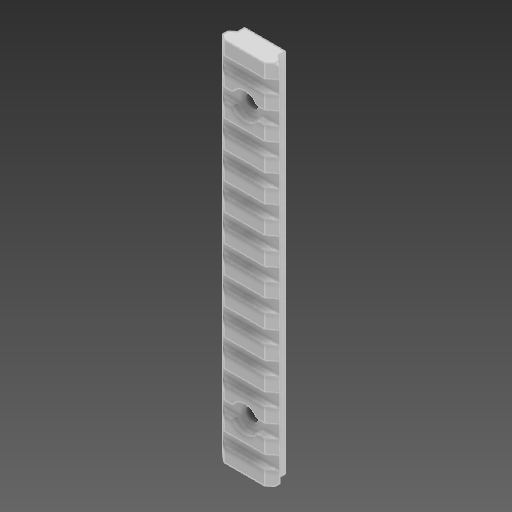
# Autodesk Inventor part: Picatinny14
Saved by Autodesk Inventor 2020.4 (Build 244396010, 396A)
## iProperties
Created: 2022-09-17
Part Number: Picatinny14
Material: Generic
Document SubType Name: Modeling
Designer: Val
Density: 1 g/cm^3
Appearance: Default
Author: Val
Autodesk Inventor part; units mm, degrees
ref_plane "YZ Plane" through (0, 0, 0) normal (1, 0, 0) x (0, 1, 0)
ref_plane "XZ Plane" through (0, 0, 0) normal (0, 1, 0) x (-1, 0, 0)
ref_plane "XY Plane" through (0, 0, 0) normal (0, 0, 1) x (1, 0, 0)
sketch "Base" plane through (0, 0, 0) normal (0, 0, 1) x (1, 0, 0)
  line L0 (-7.5, 135) -> (7.5, 135)
  line L1 (7.5, 135) -> (7.5, 0)
  line L2 (7.5, 0) -> (-7.5, 0)
  line L3 (-7.5, 0) -> (-7.5, 135)
  point P0 (0, 0)
  point P1 (0, 0)
  dimension "d0" = 135
  dimension "d1" = 15
  constraints: 8 end point, 2 parallel, 1 coincident, 1 horizontal, 1 midpoint, 1 perpendicular
  measures "d0" distance of L2.end L0.start
  measures "d1" distance of L0.start L0.end
extrude "BaseFeature" add sketch "Base" along normal blind 2.54
sketch "Profile" plane through (-7.5, 0, 0) normal (0, -1, 0) x (1, 0, 0)
  line L0 (0, 2.54) -> (15, 2.54) projected
  line L1 (0, 2.54) -> (15, 2.54)
  line L2 (15, 2.54) -> (15, 7.5692) construction
  line L3 (15, 7.5692) -> (0, 7.5692)
  line L4 (0, 7.5692) -> (0, 2.54) construction
  line L5 (-3.041, 5.0546) -> (18.041, 5.0546) construction
  line L6 (15, 7.5692) -> (18.041, 5.0546)
  line L7 (15, 2.54) -> (18.041, 5.0546)
  line L8 (0, 7.5692) -> (-3.041, 5.0546)
  line L9 (-3.041, 5.0546) -> (0, 2.54)
  point P0 (7.5, 0)
  point P1 (15, 5.0546)
  dimension "d4" = 5.0292
  dimension "d5" = 21.082
  constraints: 18 end point, 4 parallel, 2 horizontal, 1 midpoint, 1 perpendicular, 1 point on line
  measures "d4" distance of L0.end L2.end
  measures "d5" distance of L5.start L5.end
extrude "ProfileFeature" add sketch "Profile" against normal up to surface (135 mm away)
sketch "Rails" plane through (-7.5, 0, 7.5692) normal (0, 0, 1) x (1, 0, 0)
  line L0 (-3.041, 0) -> (-3.041, 135) projected
  line L1 (-3.041, 135) -> (18.041, 135)
  line L2 (18.041, 135) -> (18.041, 130)
  line L3 (18.041, 130) -> (-3.041, 130)
  line L4 (-3.041, 130) -> (-3.041, 135)
  line L5 (18.041, 0) -> (18.041, 135) projected
  line L6 (18.041, 120) -> (-3.041, 120)
  line L7 (-3.041, 125) -> (18.041, 125)
  line L8 (-3.041, 120) -> (-3.041, 125)
  line L9 (18.041, 125) -> (18.041, 120)
  line L10 (18.041, 110) -> (-3.041, 110)
  line L11 (-3.041, 115) -> (18.041, 115)
  line L12 (-3.041, 110) -> (-3.041, 115)
  line L13 (18.041, 115) -> (18.041, 110)
  line L14 (18.041, 100) -> (-3.041, 100)
  line L15 (-3.041, 105) -> (18.041, 105)
  line L16 (-3.041, 100) -> (-3.041, 105)
  line L17 (18.041, 105) -> (18.041, 100)
  line L18 (18.041, 90) -> (-3.041, 90)
  line L19 (-3.041, 95) -> (18.041, 95)
  line L20 (-3.041, 90) -> (-3.041, 95)
  line L21 (18.041, 95) -> (18.041, 90)
  line L22 (18.041, 80) -> (-3.041, 80)
  line L23 (-3.041, 85) -> (18.041, 85)
  line L24 (-3.041, 80) -> (-3.041, 85)
  line L25 (18.041, 85) -> (18.041, 80)
  line L26 (18.041, 70) -> (-3.041, 70)
  line L27 (-3.041, 75) -> (18.041, 75)
  line L28 (-3.041, 70) -> (-3.041, 75)
  line L29 (18.041, 75) -> (18.041, 70)
  line L30 (18.041, 60) -> (-3.041, 60)
  line L31 (-3.041, 65) -> (18.041, 65)
  line L32 (-3.041, 60) -> (-3.041, 65)
  line L33 (18.041, 65) -> (18.041, 60)
  line L34 (18.041, 50) -> (-3.041, 50)
  line L35 (-3.041, 55) -> (18.041, 55)
  line L36 (-3.041, 50) -> (-3.041, 55)
  line L37 (18.041, 55) -> (18.041, 50)
  line L38 (18.041, 40) -> (-3.041, 40)
  line L39 (-3.041, 45) -> (18.041, 45)
  line L40 (-3.041, 40) -> (-3.041, 45)
  line L41 (18.041, 45) -> (18.041, 40)
  line L42 (18.041, 30) -> (-3.041, 30)
  line L43 (-3.041, 35) -> (18.041, 35)
  line L44 (-3.041, 30) -> (-3.041, 35)
  line L45 (18.041, 35) -> (18.041, 30)
  line L46 (18.041, 20) -> (-3.041, 20)
  line L47 (-3.041, 25) -> (18.041, 25)
  line L48 (-3.041, 20) -> (-3.041, 25)
  line L49 (18.041, 25) -> (18.041, 20)
  line L50 (18.041, 10) -> (-3.041, 10)
  line L51 (-3.041, 15) -> (18.041, 15)
  line L52 (-3.041, 10) -> (-3.041, 15)
  line L53 (18.041, 15) -> (18.041, 10)
  line L54 (18.041, 0) -> (-3.041, 0)
  line L55 (-3.041, 5) -> (18.041, 5)
  line L56 (-3.041, 0) -> (-3.041, 5)
  line L57 (18.041, 5) -> (18.041, 0)
  point P0 (7.5, 0)
  point P1 (-3.041, 10)
  point P2 (-3.041, 20)
  point P3 (18.041, 25)
  point P4 (-3.041, 30)
  point P5 (18.041, 35)
  point P6 (18.041, 40)
  point P7 (-3.041, 40)
  point P8 (-3.041, 50)
  point P9 (-3.041, 60)
  point P10 (-3.041, 70)
  point P11 (18.041, 80)
  point P12 (-3.041, 80)
  point P13 (18.041, 85)
  point P14 (18.041, 90)
  point P15 (-3.041, 90)
  point P16 (18.041, 95)
  point P17 (18.041, 100)
  point P18 (-3.041, 100)
  point P19 (18.041, 105)
  point P20 (18.041, 110)
  point P21 (-3.041, 110)
  point P22 (18.041, 115)
  point P23 (18.041, 120)
  point P24 (-3.041, 120)
  point P25 (18.041, 125)
  point P26 (18.041, 130)
  point P27 (-3.041, 130)
  dimension "d8" = 5
  dimension "d11" = 10
  constraints: 112 end point, 52 vertical alignment, 28 parallel, 26 collinear, 1 horizontal, 1 perpendicular, 1 vertical, 2 other
  measures "d8" distance between parallel lines of L1 L3
  measures "d11" distance of L2.end L6.start
extrude "RailsFeature" cut sketch "Rails" against normal up to surface (2.5146 mm away) contours L0 L50 L5 L55 | L0 L46 L5 L51 | L0 L42 L5 L47 | L0 L38 L5 L43 | L0 L34 L5 L39 | L0 L30 L5 L35 | L0 L26 L5 L31 | L0 L22 L5 L27 | L0 L18 L5 L23 | L0 L14 L5 L19 | L0 L10 L5 L15 | L0 L6 L5 L11 | L0 L3 L5 L7
sketch "Corners" plane through (-7.5, 135, 7.5692) normal (0, 0, 1) x (1, 0, 0)
  line L0 (18.041, -130) -> (15, -130) projected
  line L1 (15, -135) -> (15, -130) projected
  line L2 (18.041, -135) -> (15, -135) projected
  line L3 (18.041, -135) -> (18.041, -130) projected
  line L4 (0, -130) -> (-3.041, -130) projected
  line L5 (-3.041, -135) -> (-3.041, -130) projected
  line L6 (0, -135) -> (-3.041, -135) projected
  line L7 (0, -135) -> (0, -130) projected
  line L8 (15, -5) -> (18.041, -5) projected
  line L9 (18.041, -5) -> (18.041, 0) projected
  line L10 (18.041, 0) -> (15, 0) projected
  line L11 (15, -5) -> (15, 0) projected
  line L12 (-3.041, -5) -> (0, -5) projected
  line L13 (0, -5) -> (0, 0) projected
  line L14 (0, 0) -> (-3.041, 0) projected
  line L15 (-3.041, -5) -> (-3.041, 0) projected
  line L16 (15, 0) -> (18.041, 0) projected
  line L17 (16.9263, 0) -> (18.041, -1.0037)
  line L18 (18.041, -5) -> (18.041, 0) projected
  line L19 (16.9263, 0) -> (18.041, 0)
  line L20 (-3.041, 0) -> (0, 0) projected
  line L21 (-3.041, 0) -> (-3.041, -1.0037)
  line L22 (-3.041, -5) -> (-3.041, 0) projected
  line L23 (-1.9263, 0) -> (-3.041, 0)
  line L24 (-3.041, -1.0037) -> (-1.9263, 0)
  line L25 (18.041, -135) -> (18.041, -130) projected
  line L26 (18.041, -135) -> (18.041, -133.8853)
  line L27 (18.041, -135) -> (17.0373, -135)
  line L28 (15, -135) -> (18.041, -135) projected
  line L29 (18.041, -133.8853) -> (17.0373, -135)
  line L30 (-3.041, -135) -> (-3.041, -133.8853)
  line L31 (-3.041, -135) -> (-3.041, -130) projected
  line L32 (-3.041, -135) -> (-2.0373, -135)
  line L33 (0, -135) -> (-3.041, -135) projected
  line L34 (-3.041, -133.8853) -> (-2.0373, -135)
  point P0 (7.5, -135)
  point P1 (-3.041, -133.8853)
  point P2 (18.041, -1.0037)
  point P3 (-3.041, -1.0037)
  dimension "d18" = 132
  dimension "d19" = 1.5
  constraints: 22 end point, 8 point on line, 6 equal length, 1 collinear, 1 perpendicular
  measures "d18" angle of L9 L17
  measures "d19" distance of L17.start L17.end
extrude "CornersFeature" cut sketch "Corners" against normal through all contours L3 L2 L29 | L34 L6 L5 | L17 L10 L9 | L15 L14 L24
sketch "MountHoles" plane through (-10.541, 120, 5.0546) normal (0, 0, 1) x (1, 0, 0)
  line L0 (0, 0) -> (21.082, 0) construction
  line L1 (0, -5) -> (0, 0) construction
  line L2 (21.082, -5) -> (0, -5) construction
  line L3 (21.082, -5) -> (21.082, 0) construction
  line L4 (0, -100) -> (21.082, -100) construction
  line L5 (0, -105) -> (0, -100) construction
  line L6 (21.082, -105) -> (0, -105) construction
  line L7 (21.082, -105) -> (21.082, -100) construction
  line L8 (21.082, -5) -> (21.082, 0) construction
  line L9 (21.082, -2.5) -> (0, -2.5) construction
  line L10 (0, -5) -> (0, 0) construction
  line L11 (21.082, -105) -> (21.082, -100) construction
  line L12 (21.082, -102.5) -> (0, -102.5) construction
  line L13 (0, -105) -> (0, -100) construction
  circle A0 centre (10.541, -102.5) radius 2.5 construction
  line L14 (18.041, -105) -> (3.041, -105) construction
  circle A1 centre (10.541, -2.5) radius 2.5 construction
  line L15 (3.041, 0) -> (18.041, 0) construction
  point P0 (10.541, -120)
  constraints: 6 midpoint, 4 end point, 2 centre point, 2 tangent
hole "MountHolesFeature" at (0, 117.5, 5.0546) at (0, 17.5, 5.0546) direction (0, 0, -1) diameter 5 depth 25.4 tip angle 118
sketch "Countersinks" plane through (-10.541, 15, 5.0546) normal (0, 0, 1) x (1, 0, 0)
  arc A0 (10.541, 0) -> (10.541, 5) centre (10.541, 2.5) ccw projected
  arc A1 (10.541, 5) -> (10.541, 0) centre (10.541, 2.5) ccw projected
  arc A2 (10.541, 100) -> (10.541, 105) centre (10.541, 102.5) ccw projected
  arc A3 (10.541, 105) -> (10.541, 100) centre (10.541, 102.5) ccw projected
  circle A4 centre (10.541, 102.5) radius 5
  circle A5 centre (10.541, 2.5) radius 5
  point P0 (10.541, -15)
  dimension "d29" = 10
  constraints: 2 centre point, 2 coincident, 1 equal radius
  measures "d29" diameter of A4
extrude "CountersinksFeature" cut sketch "Countersinks" along normal through all contours A1 A0 | A3 A2 | A4 | A5
sketch "Spacers" plane through (0, 0, 0) normal (0, 0, -1) x (-1, 0, 0)
  circle A0 centre (0, 117.5) radius 2.5 projected
  circle A1 centre (0, 17.5) radius 2.5 projected
  circle A2 centre (0, 117.5) radius 2.5 projected
  circle A3 centre (0, 117.5) radius 3.5
  circle A4 centre (0, 17.5) radius 2.5 projected
  circle A5 centre (0, 17.5) radius 3.5
  point P0 (0, 0)
  dimension "d32" = 1
  constraints: 2 centre point, 2 coincident, 1 equal radius
  measures "d32" radial gap between concentric circles of A3 A0
extrude "SpacersFeature" add sketch "Spacers" along normal blind 1
body "Solid1"
